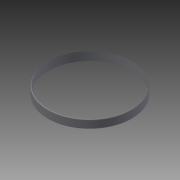
# Autodesk Inventor part: Prop_Ring
Saved by Autodesk Inventor 2015 (Build 190159000, 159)
## iProperties
Created: 2016-03-22
Part Number: Prop_Ring
Material: Generic
Document SubType Name: Modeling
Designer: 839364
Density: 1 g/cm^3
Appearance: Default
Author: 839364
Autodesk Inventor part; units mm, degrees
ref_plane "YZ Plane" through (0, 0, 0) normal (1, 0, 0) x (0, 1, 0)
ref_plane "XZ Plane" through (0, 0, 0) normal (0, 1, 0) x (-1, 0, 0)
ref_plane "XY Plane" through (0, 0, 0) normal (0, 0, 1) x (1, 0, 0)
sketch "Sketch1" plane through (0, 0, 0) normal (0, 1, 0) x (-1, 0, 0)
  circle A0 centre (0, 0) radius 125.73
  circle A1 centre (0, 0) radius 127
  dimension "d0" = 251.46
  dimension "d1" = 254
  constraints: 2 centre point, 2 coincident
  measures "d0" diameter of A0
  measures "d1" diameter of A1
extrude "Extrusion1" add sketch "Sketch1" along normal blind 25.4
fillet "Fillet1" radius 3.175 1 edges at (127, 25.4, 0)
fillet "Fillet2" radius 3.175 1 edges at (127, 0, 0)
body "Solid1"
